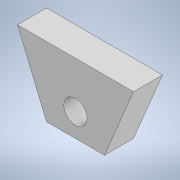
# Autodesk Inventor part: N2
Saved by Autodesk Inventor 2022 (Build 260153000, 153)
## iProperties
Created: 2023-03-30
Part Number: N2
Material: Типовые
Document SubType Name: Modeling
Designer: Hp
Density: 1 g/cm^3
Appearance: По умолчанию
Author: Hp
Autodesk Inventor part; units mm, degrees
ref_plane "YZ Plane" through (0, 0, 0) normal (1, 0, 0) x (0, 1, 0)
ref_plane "XZ Plane" through (0, 0, 0) normal (0, 1, 0) x (-1, 0, 0)
ref_plane "XY Plane" through (0, 0, 0) normal (0, 0, 1) x (1, 0, 0)
sketch "Эскиз1" plane through (0, 0, 0) normal (0, 0, 1) x (1, 0, 0)
  line L0 (10, 0) -> (30, 0)
  line L1 (30, 0) -> (40, 24)
  line L2 (10, 0) -> (0, 24)
  circle A0 centre (20, 8) radius 4
  line L3 (0, 24) -> (40, 24)
  point P0 (0, 0)
  dimension "d0" = 24
  dimension "d1" = 40
  dimension "d3" = 20
  dimension "d6" = 8
  constraints: 8 end point, 1 centre point, 1 horizontal
  measures "d0" distance of point (0, 0) L2.end
  measures "d1" distance of L2.end L1.end
  measures "d3" distance of L0.start L0.end
  measures "d6" diameter of A0
extrude "Выдавливание1" add sketch "Эскиз1" along normal blind 10
